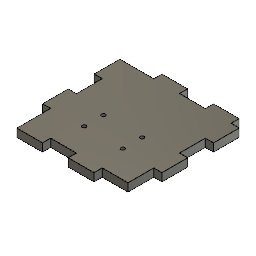
Front (Autodesk Fusion 360 design; units mm, degrees)
Autodesk Fusion 360 part; units mm, degrees
sketch "Sketch1" plane through (0, 0, 0) normal (0, 1, 0) x (1, 0, 0)
  circle A0 centre (25, 21) radius 1.5
  circle A1 centre (25, 36) radius 1.5
  circle A2 centre (55, 21) radius 1.5
  circle A3 centre (55, 36) radius 1.5
  line L0 (20, 0) -> (20, -6.35)
  line L1 (20, -6.35) -> (0, -6.35)
  line L2 (0, -6.35) -> (0, 0)
  line L3 (60, 0) -> (60, -6.35)
  line L4 (60, -6.35) -> (40, -6.35)
  line L5 (40, -6.35) -> (40, 0)
  line L6 (80, 20) -> (86.35, 20)
  line L7 (86.35, 20) -> (86.35, 40)
  line L8 (86.35, 40) -> (80, 40)
  line L9 (80, 60) -> (86.35, 60)
  line L10 (86.35, 60) -> (86.35, 80)
  line L11 (86.35, 80) -> (80, 80)
  line L12 (0, 20) -> (-6.35, 20)
  line L13 (-6.35, 20) -> (-6.35, 40)
  line L14 (-6.35, 40) -> (0, 40)
  line L15 (0, 60) -> (-6.35, 60)
  line L16 (-6.35, 60) -> (-6.35, 80)
  line L17 (-6.35, 80) -> (0, 80)
  line L18 (60, 80) -> (60, 86.35)
  line L19 (60, 86.35) -> (80, 86.35)
  line L20 (80, 86.35) -> (80, 80)
  line L21 (20, 80) -> (20, 86.35)
  line L22 (20, 86.35) -> (40, 86.35)
  line L23 (40, 86.35) -> (40, 80)
  line L24 (20, 0) -> (20, -6.35)
  line L25 (20, -6.35) -> (0, -6.35)
  line L26 (0, -6.35) -> (0, 0)
  line L27 (20, 0) -> (40, 0)
  line L28 (40, 0) -> (40, -6.35)
  line L29 (40, -6.35) -> (60, -6.35)
  line L30 (60, -6.35) -> (60, 0)
  line L31 (60, 0) -> (80, 0)
  line L32 (80, 0) -> (80, 20)
  line L33 (80, 20) -> (86.35, 20)
  line L34 (86.35, 20) -> (86.35, 40)
  line L35 (86.35, 40) -> (80, 40)
  line L36 (80, 40) -> (80, 60)
  line L37 (80, 60) -> (86.35, 60)
  line L38 (86.35, 60) -> (86.35, 80)
  line L39 (86.35, 80) -> (80, 80)
  line L40 (80, 80) -> (80, 86.35)
  line L41 (80, 86.35) -> (60, 86.35)
  line L42 (60, 86.35) -> (60, 80)
  line L43 (60, 80) -> (40, 80)
  line L44 (40, 80) -> (40, 86.35)
  line L45 (40, 86.35) -> (20, 86.35)
  line L46 (20, 86.35) -> (20, 80)
  line L47 (20, 80) -> (-6.35, 80)
  line L48 (-6.35, 80) -> (-6.35, 60)
  line L49 (-6.35, 60) -> (0, 60)
  line L50 (0, 60) -> (0, 40)
  line L51 (0, 40) -> (-6.35, 40)
  line L52 (-6.35, 40) -> (-6.35, 20)
  line L53 (-6.35, 20) -> (0, 20)
  line L54 (0, 20) -> (0, 0)
  dimension "d2" = 80
  dimension "d3" = 3
  dimension "d4" = 3
  dimension "d5" = 3
  dimension "d6" = 3
  dimension "d8" = 15
  dimension "d10" = 15
  dimension "d11" = 30
  dimension "d12" = 30
  dimension "d19" = 6.35
  dimension "d20" = 20
  dimension "d21" = 6.35
  dimension "d22" = 20
  dimension "d23" = 20
  dimension "d24" = 6.35
  dimension "d26" = 20
  dimension "d27" = 20
  dimension "d28" = 6.35
  dimension "d29" = 20
  dimension "d30" = 6.35
  dimension "d31" = 20
  dimension "d32" = 6.35
  dimension "d33" = 20
  dimension "d34" = 20
  dimension "d36" = 6.35
  dimension "d37" = 20
  dimension "d38" = 6.35
  dimension "d39" = 20
  dimension "d40" = 20
  measures "d3" diameter of A0
  measures "d4" diameter of A1
  measures "d5" diameter of A2
  measures "d6" diameter of A3
  measures "d19" distance of L2.end
  measures "d21" distance of L2.end
  measures "d23" distance of L0 L5
  measures "d29" distance of L8 L9
  measures "d34" distance of L14 L15
  measures "d40" distance of L18 L23
extrude "Extrude3" add sketch "Sketch1" along normal blind 6.35
extrude "Extrude2" [suppressed]
extrude "Extrude1" [suppressed]
equation "height = 75 mm" comment "Height of the front"
equation "Acryllic_thickness = 6.35 mm"
